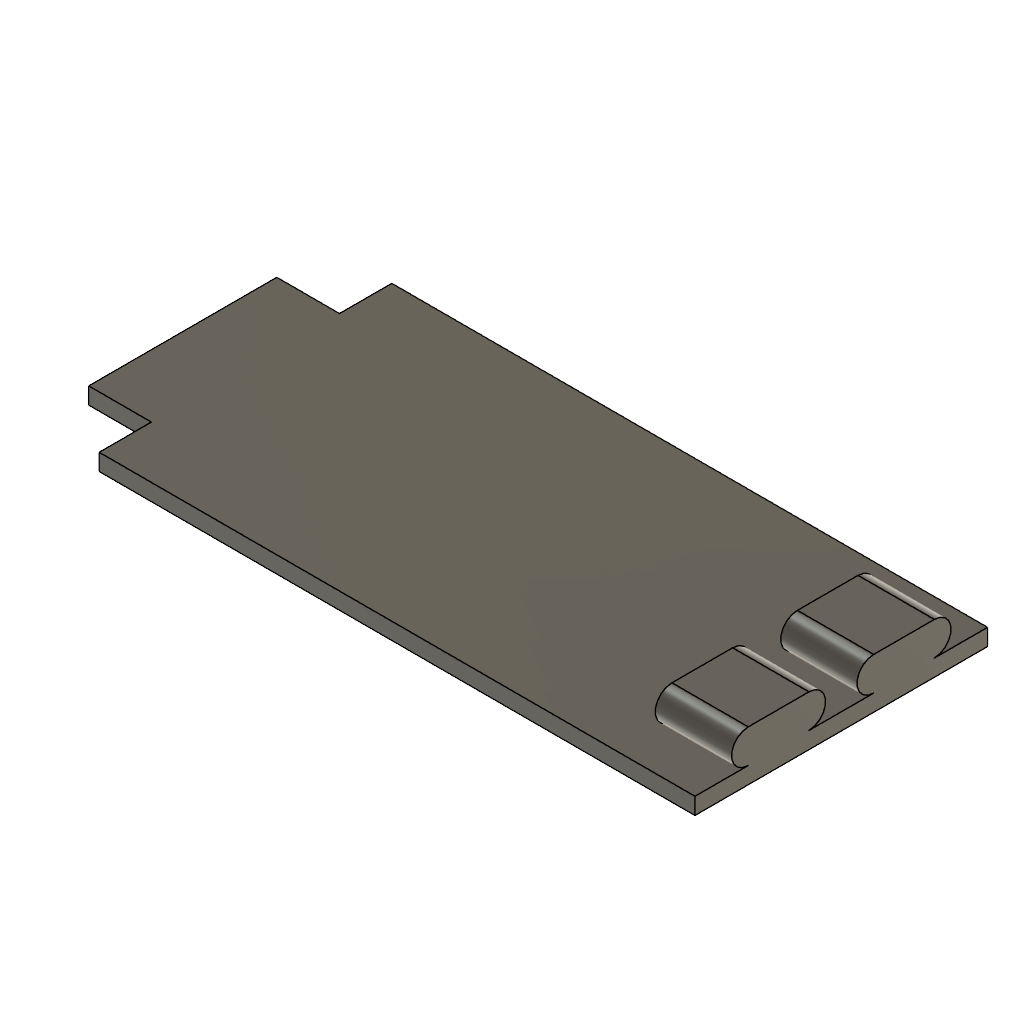
ESP32-S3 (Autodesk Fusion 360 design; units mm, degrees)
Autodesk Fusion 360 part; units mm, degrees
sketch "Skizze1" plane through (0, 0, 0) normal (0, 0, 1) x (1, 0, 0)
  line L0 (0, 0) -> (-57, 0)
  line L1 (-57, 0) -> (-57, 28)
  line L2 (-57, 28) -> (0, 28)
  line L3 (0, 28) -> (0, 0)
  line L4 (-57, 23) -> (-63, 23)
  line L5 (-63, 23) -> (-63, 5)
  line L6 (-63, 5) -> (-57, 5)
  line L7 (-57, 5) -> (-57, 23)
  line L8 (0, 14) -> (-57, 14) construction
  dimension "d1" = 57
  dimension "d2" = 28
  dimension "d3" = 6
  dimension "d4" = 18
  constraint horizontal L0
  constraint vertical L1
  constraint horizontal L2
  constraint vertical L3
  constraint coincident L0.start L3.end
  constraint horizontal L4
  constraint vertical L5
  constraint horizontal L6
  constraint vertical L7
  constraint coincident L1 L4.start
  constraint midpoint L3 L8.start
  constraint coincident L1 L8.end
  constraint horizontal L8
  constraint symmetric L4 L6 L8
  measures "d1" distance of L1.end L2.end
  measures "d2" distance of L0.end L1.end
  measures "d3" distance of L4.start L4.end
  measures "d4" distance of L4.end L6
extrude "Extrusion1" add sketch "Skizze1" along normal blind 1.6
sketch "Skizze2" plane through (0, 0, 0) normal (1, 0, 0) x (0, 1, 0)
  line L0 (0, 0) -> (28, 0)
  line L1 (28, 0) -> (28, 1.6)
  line L2 (28, 1.6) -> (0, 1.6)
  line L3 (0, 1.6) -> (0, 0)
  line L4 (23, 1.6) -> (5, 1.6)
  line L5 (5, 1.6) -> (0, 1.6)
  line L6 (0, 1.6) -> (28, 1.6)
  line L7 (28, 1.6) -> (23, 1.6)
  line L8 (5.1, 4.8) -> (10.9, 4.8)
  line L9 (10.9, 1.6) -> (5.1, 1.6)
  line L10 (17.1, 4.8) -> (22.9, 4.8)
  line L11 (17.1, 1.6) -> (22.9, 1.6)
  arc A0 (5.1, 4.8) -> (5.1, 1.6) centre (5.1, 3.2) ccw
  arc A1 (10.9, 1.6) -> (10.9, 4.8) centre (10.9, 3.2) ccw
  arc A2 (17.1, 4.8) -> (17.1, 1.6) centre (17.1, 3.2) ccw
  arc A3 (22.9, 1.6) -> (22.9, 4.8) centre (22.9, 3.2) ccw
  line L12 (14, 1.6) -> (14, 0) construction
  dimension "d7" = 3.2
  dimension "d8" = 3.2
  dimension "d9" = 5.8
  dimension "d10" = 5.8
  dimension "d11" = 6.2
  constraint horizontal L10
  constraint horizontal L11
  constraint horizontal L8
  constraint horizontal L9
  constraint tangent L10 A3
  constraint tangent L10 A2
  constraint tangent L11 A2
  constraint tangent L11 A3
  constraint tangent L8 A1
  constraint tangent L8 A0
  constraint tangent L9 A0
  constraint tangent L9 A1
  constraint coincident L6 L9.start
  constraint coincident L2 L11.start
  constraint midpoint L6 L12.start
  constraint midpoint L0 L12.end
  constraint symmetric L9.start L11.start L12
  measures "d7" distance of L10 L11
  measures "d8" distance of L8 L9
  measures "d9" distance of A0.centre A1.centre
  measures "d10" distance of A2.centre A3.centre
  measures "d11" distance of A1.centre A2.centre
extrude "Extrusion2" add sketch "Skizze2" against normal blind 7.3 contours L2 L4 L6 L8 L9 A0 A1 | L2 L4 L6 L10 L11 A2 A3
sketch "Skizze3" plane through (0, 0, 0) normal (0, 0, -1) x (1, 0, 0)
  line L0 (-63, -23) -> (-57, -23)
  line L1 (-57, -23) -> (-57, -28)
  line L2 (-57, -28) -> (0, -28)
  line L3 (0, -28) -> (0, 0)
  line L4 (0, 0) -> (-57, 0)
  line L5 (-57, 0) -> (-57, -5)
  line L6 (-57, -5) -> (-63, -5)
  line L7 (-63, -5) -> (-63, -23)
  line L8 (0, -26.7) -> (-57, -26.7) construction
  line L9 (0, -1.3) -> (-57, -1.3) construction
  line L10 (-1.83, -26.7) -> (-1.83, -1.3) construction
  line L11 (-55.17, -26.7) -> (-55.17, -1.3) construction
  line L12 (-1.83, -26.7) -> (0, -26.7) construction
  line L13 (-57, -26.7) -> (-55.17, -26.7) construction
  line L14 (0, -14) -> (-63, -14) construction
  point P0 (-1.83, -1.3)
  point P1 (-55.17, -1.3)
  point P2 (-55.17, -26.7)
  point P3 (-1.83, -26.7)
  dimension "d14" = 53.34
  dimension "d16" = 25.4
  constraint coincident L3 L8.start
  constraint coincident L1 L8.end
  constraint coincident L3 L9.start
  constraint coincident L5 L9.end
  constraint horizontal L9
  constraint horizontal L8
  constraint coincident L9 P0
  constraint coincident L9 P1
  constraint coincident L8 P2
  constraint coincident L8 P3
  constraint coincident P3 L10.start
  constraint coincident P2 L11.start
  constraint vertical L10
  constraint vertical L11
  constraint coincident P0 L10.end
  constraint coincident P1 L11.end
  constraint equal L12 L13
  constraint midpoint L3 L14.start
  constraint midpoint L7 L14.end
  constraint symmetric P0 P3 L14
  measures "d14" distance of L10 L11
  measures "d16" distance of L8 L9
equation "d8 = d7"
equation "d9 = d10"
equation "d10 = 9 mm - 3.2 mm"
equation "d11 = 3 mm + 3.2 mm"
equation "d14 = ( 21 * 2.54 ) * 1 mm"
equation "d16 = ( 10 * 2.54 ) * 1 mm"
